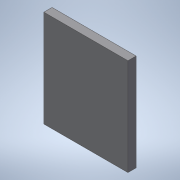
# Autodesk Inventor part: belt circufrence
Saved by Autodesk Inventor 2020 (Build 240168000, 168)
## iProperties
Created: 2019-05-26
Part Number: belt circufrence
Material: Generic
Document SubType Name: Modeling
Designer: LillaHunden
Density: 1 g/cm^3
Appearance: Default
Author: LillaHunden
Autodesk Inventor part; units mm, degrees
ref_plane "YZ Plane" through (0, 0, 0) normal (1, 0, 0) x (0, 1, 0)
ref_plane "XZ Plane" through (0, 0, 0) normal (0, 1, 0) x (-1, 0, 0)
ref_plane "XY Plane" through (0, 0, 0) normal (0, 0, 1) x (1, 0, 0)
sketch "Sketch1" plane through (0, 0, 0) normal (0, 0, 1) x (1, 0, 0)
  line L0 (-219.6419, 61.3316) -> (-117.215, 61.3316)
  line L1 (-117.215, 61.3316) -> (-117.215, -56.6617)
  line L2 (-117.215, -56.6617) -> (-219.6419, -56.6617)
  line L3 (-219.6419, -56.6617) -> (-219.6419, 61.3316)
  point P0 (0, 0)
  constraints: 8 end point, 2 parallel, 1 horizontal, 1 perpendicular
extrude "Extrusion1" add sketch "Sketch1" along normal blind 10
sketch "Sketch2" plane through (0, 0, 10) normal (0, 0, 1) x (1, 0, 0)
  line L0 (-165.5966, 48.7171) -> (-165.5966, -16.2829) construction
  line L1 (-171.5966, 42.7171) -> (-171.5966, -10.2829)
  line L2 (-159.5966, -10.2829) -> (-159.5966, 42.7171)
  arc A0 (-159.5966, 42.7171) -> (-171.5966, 42.7171) centre (-165.5966, 42.7171) ccw
  arc A1 (-171.5966, -10.2829) -> (-159.5966, -10.2829) centre (-165.5966, -10.2829) ccw
  point P0 (0, 0)
  point P1 (-165.5966, 16.2171)
  dimension "d2" = 12
  dimension "d3" = 65
  constraints: 8 end point, 6 point on circle, 4 tangent, 2 centre point, 2 point on line, 1 midpoint, 1 parallel, 1 vertical
  measures "d2" diameter of A1
  measures "d3" distance of L0.start L0.end
extrude "Extrusion2" cut sketch "Sketch2" against normal through all
body "Solid1"
